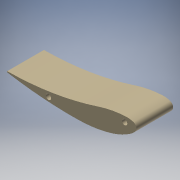
# Autodesk Inventor part: uretan_s
Saved by Autodesk Inventor 2018 (Build 220112000, 112)
## iProperties
Created: 2018-04-20
Part Number: uretan_s
Material: ポリエチレン、高密度
Document SubType Name: Modeling
Designer: ku_sk
Density: 0.952 g/cm^3
Appearance: ベージュ
Author: ku_sk
Autodesk Inventor part; units mm, degrees
ref_plane "YZ Plane" through (0, 0, 0) normal (1, 0, 0) x (0, 1, 0)
ref_plane "XZ Plane" through (0, 0, 0) normal (0, 1, 0) x (-1, 0, 0)
ref_plane "XY Plane" through (0, 0, 0) normal (0, 0, 1) x (1, 0, 0)
sketch "スケッチ1" plane through (0, 0, 0) normal (0, 1, 0) x (-1, 0, 0)
  arc A0 (72.9254, -25.3463) -> (139.4294, -19.0858) centre (64.9013, 416.2515) ccw projected
  arc A1 (54.1052, -25.1311) -> (72.9254, -25.3463) centre (67.1484, 292.5868) ccw projected
  arc A2 (19.6951, -19.0145) -> (54.1052, -25.1311) centre (59.4352, 104.7024) ccw projected
  arc A3 (-0.0609, -9.311) -> (19.6951, -19.0145) centre (42.8692, 53.13) ccw projected
  arc A4 (-5.5029, -4.0266) -> (-0.0609, -9.311) centre (12.76, 9.3368) ccw projected
  arc A5 (-2.9938, 3.6874) -> (-5.5029, -4.0266) centre (-1.4678, -1.074) ccw projected
  arc A6 (5.1717, 4.7562) -> (-2.9938, 3.6874) centre (4.0256, -18.2153) ccw projected
  arc A7 (36.109, -0.9508) -> (5.1717, 4.7562) centre (-0.7578, -114.096) ccw projected
  arc A8 (36.109, -0.9508) -> (38.0145, -1.5673) centre (185.125, 456.3841) ccw projected
  arc A9 (38.0145, -1.5673) -> (139.3334, -17.8944) centre (142.307, 323.0926) ccw projected
  arc A10 (139.4294, -19.0858) -> (139.3334, -17.8944) centre (139.3282, -18.4944) ccw projected
  circle A11 centre (6.8478, -1.4519) radius 3 projected
  circle A12 centre (92.934, -19.7045) radius 3 projected
  point P0 (0, 0)
extrude "押し出し1" add sketch "スケッチ1" along normal mid plane 41.5
